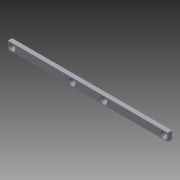
# Autodesk Inventor part: Protector
Saved by Autodesk Inventor 2012 (Build 160160000, 160)
## iProperties
Created: 2012-04-10
Part Number: Protector
Material: Aluminum-6061
Document SubType Name: Modeling
Designer: admin
Density: 2.71 g/cm^3
Mass: 24.3311 g
Surface Area: 59.2556 cm^2
Volume: 8.97828 cm^3
Author: admin
Autodesk Inventor part; units mm, degrees
ref_plane "YZ Plane" through (0, 0, 0) normal (1, 0, 0) x (0, 1, 0)
ref_plane "XZ Plane" through (0, 0, 0) normal (0, 1, 0) x (-1, 0, 0)
ref_plane "XY Plane" through (0, 0, 0) normal (0, 0, 1) x (1, 0, 0)
sketch "Sketch1" plane through (0, 0, 0) normal (0, 0, 1) x (1, 0, 0)
  line L0 (0, 0) -> (195.58, 0)
  line L1 (195.58, 0) -> (195.58, 9.525)
  line L2 (195.58, 9.525) -> (0, 9.525)
  line L3 (0, 9.525) -> (0, 0)
  dimension "d0" = 195.58
  dimension "d1" = 9.525
  constraints: 8 end point, 2 parallel, 1 horizontal, 1 perpendicular
  measures "d0" distance between parallel lines of L1 L3
  measures "d1" distance between parallel lines of L2 L0
extrude "Extrusion1" add sketch "Sketch1" along normal blind 5.08
sketch "Sketch2" plane through (0, 0, 5.08) normal (0, 0, 1) x (1, 0, 0)
  line L0 (195.58, 0) -> (0, 0) projected
  line L1 (0, 9.525) -> (195.58, 9.525) projected
  line L2 (0, 36.0407) -> (9.525, 36.0407) projected
  line L3 (0, -27.6521) -> (0, 36.0407) projected
  line L4 (9.525, -27.6521) -> (0, -27.6521) projected
  line L5 (9.525, 36.0407) -> (9.525, -27.6521) projected
  line L6 (195.58, -24.7204) -> (195.58, 5.4842) projected
  line L7 (195.58, -24.7204) -> (186.055, -24.7204) projected
  line L8 (186.055, 5.4842) -> (186.055, -24.7204) projected
  line L9 (186.055, 5.4842) -> (195.58, 5.4842) projected
  line L10 (83.185, 2.2202) -> (73.66, 2.2202) projected
  line L11 (73.66, 2.2202) -> (73.66, -16.2449) projected
  line L12 (83.185, -16.2449) -> (73.66, -16.2449) projected
  line L13 (83.185, -16.2449) -> (83.185, 2.2202) projected
  line L14 (112.395, 2.2202) -> (121.92, 2.2202) projected
  line L15 (112.395, -16.2449) -> (112.395, 2.2202) projected
  line L16 (112.395, -16.2449) -> (121.92, -16.2449) projected
  line L17 (121.92, 2.2202) -> (121.92, -16.2449) projected
  line L18 (9.525, 0) -> (0, 0)
  line L19 (0, 0) -> (0, 9.525)
  line L20 (0, 9.525) -> (9.525, 9.525)
  line L21 (9.525, 9.525) -> (9.525, 0)
  line L22 (73.66, 0) -> (83.185, 0)
  line L23 (83.185, 0) -> (83.185, 9.525)
  line L24 (83.185, 9.525) -> (73.66, 9.525)
  line L25 (73.66, 9.525) -> (73.66, 0)
  line L26 (112.395, 0) -> (121.92, 0)
  line L27 (121.92, 0) -> (121.92, 9.525)
  line L28 (121.92, 9.525) -> (112.395, 9.525)
  line L29 (112.395, 9.525) -> (112.395, 0)
  line L30 (186.055, 0) -> (195.58, 0)
  line L31 (195.58, 0) -> (195.58, 9.525)
  line L32 (195.58, 9.525) -> (186.055, 9.525)
  line L33 (186.055, 9.525) -> (186.055, 0)
  point P0 (4.7625, 4.7625)
  point P1 (78.4225, 4.7625)
  point P2 (117.1575, 4.7625)
  point P3 (190.8175, 4.7625)
  constraints: 32 end point, 10 point on line, 8 parallel, 4 horizontal, 4 perpendicular
hole "Hole1" at (4.7625, 4.7625, 5.08) at (78.4225, 4.7625, 5.08) at (117.1575, 4.7625, 5.08) at (190.8175, 4.7625, 5.08) direction (0, 0, -1) diameter 4.4958 end through all countersink diameter 8.4328 countersink angle 82 clearance for "Flat Head Machine Screw (82)" size "#8" standard "Ansi Unified Screw Threads"
body "Solid1"
